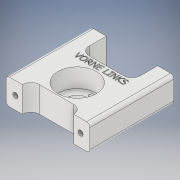
# Autodesk Inventor part: Motorhalterung leicht VL
Saved by Autodesk Inventor 2018 (Build 220112000, 112)
## iProperties
Created: 2019-03-03
Part Number: Motorhalterung leicht VL
Material: ABS-Kunststoff
Document SubType Name: Modeling
Designer: RedBots
Density: 0.513105 g/cm^3
Appearance: Weiß
Mass: 11 g
Surface Area: 84.958 cm^2
Volume: 21.4381 cm^3
Author: RedBots
Autodesk Inventor part; units mm, degrees
ref_plane "YZ Plane" through (0, 0, 0) normal (1, 0, 0) x (0, 1, 0)
ref_plane "XZ Plane" through (0, 0, 0) normal (0, 1, 0) x (-1, 0, 0)
ref_plane "XY Plane" through (0, 0, 0) normal (0, 0, 1) x (1, 0, 0)
sketch "Skizze2" plane through (0, 0, 0) normal (0, 0, 1) x (1, 0, 0)
  line L0 (0, 0) -> (49, 0)
  line L1 (0, 0) -> (49, 0) construction
  line L2 (49, 0) -> (49, 49)
  line L3 (49, 49) -> (0, 49)
  line L4 (0, 49) -> (0, 0)
  dimension "d16" = 49
  dimension "d18" = 49
  constraints: 10 end point, 2 equal length, 2 horizontal, 2 perpendicular
  measures "d16" distance of L0.start L0.end
  measures "d18" distance of L0.end L2.end
extrude "Extrusion1" add sketch "Skizze2" along normal blind 15
sketch "Skizze3" plane through (0, 0, 15) normal (0, 0, 1) x (1, 0, 0)
  circle A0 centre (24.5, 17) radius 11.25
  line L0 (0, 49) -> (0, 0) construction
  line L1 (0, 17) -> (49, 17) construction
  line L2 (49, 0) -> (49, 49) construction
  line L3 (0, 0) -> (49, 0) construction
  dimension "d72" = 22.5
  dimension "d73" = 17
  constraints: 2 end point, 2 point on line, 1 centre point, 1 coincident, 1 horizontal, 1 midpoint
  measures "d72" diameter of A0
  measures "d73" distance between parallel lines of L3 L1
extrude "Extrusion2" cut sketch "Skizze3" against normal blind 11
sketch "Skizze4" plane through (24.5, 17, 4) normal (0, 0, 1) x (1, 0, 0)
  circle A0 centre (7.3612, -4.25) radius 1.5
  circle A1 centre (0, 8.5) radius 1.5
  circle A2 centre (-7.3612, -4.25) radius 1.5
  line L0 (0, 0) -> (0, 8.5) construction
  line L1 (-24.5, -17) -> (24.5, -17) construction
  circle A3 centre (0, 0) radius 11.25 construction
  line L2 (0, -17) -> (0, 0) construction
  line L3 (0, 0) -> (7.3612, -4.25) construction
  line L4 (0, 0) -> (-7.3612, -4.25) construction
  circle A4 centre (0, 0) radius 6.5
  dimension "d37" = 3
  dimension "d42" = 3
  dimension "d43" = 3
  dimension "d90" = 8.5
  dimension "d91" = 120
  dimension "d92" = 120
  dimension "d93" = 13
  constraints: 8 end point, 4 centre point, 4 coincident, 2 equal length, 2 vertical, 1 midpoint
  measures "d37" diameter of A0
  measures "d42" diameter of A1
  measures "d43" diameter of A2
  measures "d90" distance of L0.start L0.end
  measures "d91" angle of L3 L0
  measures "d92" angle of L0 L4
  measures "d93" diameter of A4
extrude "Extrusion3" cut sketch "Skizze4" against normal up to next
sketch "Skizze9" plane through (0, 49, 0) normal (0, 1, 0) x (1, 0, 0)
  line L0 (24.5, -7.5) -> (43.5, -7.5) construction
  circle A0 centre (5.5, -7.5) radius 1.5
  circle A1 centre (43.5, -7.5) radius 1.5
  line L1 (0, -15) -> (49, -15) construction
  line L2 (24.5, -15) -> (24.5, 0) construction
  line L3 (49, 0) -> (0, 0) construction
  line L4 (5.5, -7.5) -> (24.5, -7.5) construction
  dimension "d58" = 3
  dimension "d89" = 19
  constraints: 7 end point, 3 midpoint, 2 centre point, 2 collinear, 1 coincident, 1 equal radius, 1 horizontal, 1 vertical
  measures "d58" diameter of A0
  measures "d89" distance of L0.start L0.end
extrude "Extrusion6" cut sketch "Skizze9" against normal blind 56
sketch "Skizze12" plane through (0, 0, 0) normal (0, 0, -1) x (-1, 0, 0)
  circle A0 centre (-24.5, 25.5) radius 1.5 projected
  circle A1 centre (-24.5, 25.5) radius 3
  circle A2 centre (-17.1388, 12.75) radius 1.5 projected
  circle A3 centre (-17.1388, 12.75) radius 3
  circle A4 centre (-31.8612, 12.75) radius 1.5 projected
  circle A5 centre (-31.8612, 12.75) radius 3
  point P0 (0, 0)
  dimension "d80" = 6
  dimension "d81" = 6
  dimension "d82" = 6
  constraints: 3 centre point, 3 coincident
  measures "d80" diameter of A1
  measures "d81" diameter of A3
  measures "d82" diameter of A5
extrude "Extrusion8" cut sketch "Skizze12" against normal blind 0.16
chamfer "Fase3" distance 1.5 angle 45 3 edges at (23, 25.5, 0.16) (30.3612, 12.75, 0.16) (15.6388, 12.75, 0.16)
fillet "Rundung2" radius 0.5 3 edges at (23, 25.5, 1.66) (30.3612, 12.75, 1.66) (15.6388, 12.75, 1.66)
sketch "Skizze14" plane through (0, 0, 0) normal (0, 0, -1) x (-1, 0, 0)
  line L0 (-39.5, 49) -> (-9.5, 49)
  line L1 (-9.5, 49) -> (-9.5, 34)
  line L2 (-9.5, 34) -> (-39.5, 34)
  line L3 (-39.5, 34) -> (-39.5, 49)
  line L4 (-49, 49) -> (0, 49) projected
  line L5 (-49, 0) -> (-49, 49) construction
  line L6 (0, 49) -> (0, 0) construction
  line L7 (-39.5, 0) -> (-9.5, 0)
  line L8 (-9.5, 0) -> (-9.5, 5)
  line L9 (-9.5, 5) -> (-39.5, 5)
  line L10 (-39.5, 5) -> (-39.5, 0)
  line L11 (0, 0) -> (-49, 0) projected
  point P0 (-24.5, 49)
  point P1 (-24.5, 0)
  point P2 (-24.5, 0)
  dimension "d95" = 15
  dimension "d96" = 30
  dimension "d101" = 5
  constraints: 16 end point, 6 midpoint, 3 horizontal, 3 parallel, 2 vertical, 1 perpendicular
  measures "d95" distance of L0.end L1.end
  measures "d96" distance between parallel lines of L1 L3
  measures "d101" distance of L7.end L9.start
extrude "Extrusion9" cut sketch "Skizze14" against normal up to next
fillet "Rundung3" radius 5 4 edges at (39.5, 34, 7.5) (9.5, 34, 7.5) (39.5, 5, 7.5) (9.5, 5, 7.5)
fillet "Rundung4" radius 2 4 edges at (49, 24.5, 15) (49, 24.5, 0) (0, 24.5, 0) (0, 24.5, 15)
sketch "Skizze15" plane through (0, 0, 15) normal (0, 0, 1) x (1, 0, 0)
  line L0 (34.5, 34) -> (14.5, 34) construction
  line L1 (24.5, 34) -> (24.5, 28.25) construction
  circle A0 centre (24.5, 17) radius 11.25 construction
  line L2 (12.5946, 32.875) -> (11.3892, 29.375)
  line L3 (11.3892, 29.375) -> (10.8872, 29.375)
  line L4 (10.8872, 29.375) -> (9.6817, 32.875)
  line L5 (9.6817, 32.875) -> (10.1809, 32.875)
  line L6 (10.1809, 32.875) -> (11.1509, 29.9678)
  line L7 (11.1509, 29.9678) -> (12.1209, 32.875)
  line L8 (12.1209, 32.875) -> (12.5946, 32.875)
  spline S0 degree 2 poles (15.4054, 32.4751) (15.6039, 32.2425) (15.8252, 31.5618) (15.8252, 31.125) knots 0 0 0 1 2 2 2
  spline S1 degree 2 poles (15.8252, 31.125) (15.8252, 30.6996) (15.6096, 30.0103) (15.4054, 29.7778) knots 0 0 0 1 2 2 2
  spline S2 degree 2 poles (15.4054, 29.7778) (15.1898, 29.5338) (14.6197, 29.3013) (14.2765, 29.3013) knots 0 0 0 1 2 2 2
  spline S3 degree 2 poles (14.2765, 29.3013) (13.922, 29.3013) (13.3547, 29.5423) (13.1477, 29.7778) knots 0 0 0 1 2 2 2
  spline S4 degree 2 poles (13.1477, 29.7778) (12.9463, 30.0103) (12.7308, 30.6939) (12.7308, 31.125) knots 0 0 0 1 2 2 2
  spline S5 degree 2 poles (12.7308, 31.125) (12.7308, 31.5646) (12.9491, 32.234) (13.1505, 32.4751) knots 0 0 0 1 2 2 2
  spline S6 degree 2 poles (13.1505, 32.4751) (13.3547, 32.7077) (13.9248, 32.9487) (14.2765, 32.9487) knots 0 0 0 1 2 2 2
  spline S7 degree 2 poles (14.2765, 32.9487) (14.6339, 32.9487) (15.2068, 32.6991) (15.4054, 32.4751) knots 0 0 0 1 2 2 2
  spline S8 degree 2 poles (15.3402, 31.125) (15.3402, 31.471) (15.1898, 32.0071) (15.0537, 32.1829) knots 0 0 0 1 2 2 2
  spline S9 degree 2 poles (15.0537, 32.1829) (14.9147, 32.3645) (14.5233, 32.546) (14.2794, 32.546) knots 0 0 0 1 2 2 2
  spline S10 degree 2 poles (14.2794, 32.546) (14.0269, 32.546) (13.6469, 32.3701) (13.5022, 32.1829) knots 0 0 0 1 2 2 2
  spline S11 degree 2 poles (13.5022, 32.1829) (13.3632, 32.0043) (13.2158, 31.4654) (13.2158, 31.125) knots 0 0 0 1 2 2 2
  spline S12 degree 2 poles (13.2158, 31.125) (13.2158, 30.4358) (13.7944, 29.704) (14.2794, 29.704) knots 0 0 0 1 2 2 2
  spline S13 degree 2 poles (14.2794, 29.704) (14.7644, 29.704) (15.3402, 30.4358) (15.3402, 31.125) knots 0 0 0 1 2 2 2
  line L9 (19.0444, 29.375) -> (18.4402, 29.375)
  line L10 (18.4402, 29.375) -> (17.3341, 30.7676)
  line L11 (17.3341, 30.7676) -> (16.8008, 30.7676)
  line L12 (16.8008, 30.7676) -> (16.8008, 29.375)
  line L13 (16.8008, 29.375) -> (16.3357, 29.375)
  line L14 (16.3357, 29.375) -> (16.3357, 32.875)
  line L15 (16.3357, 32.875) -> (17.2376, 32.875)
  spline S14 degree 2 poles (17.2376, 32.875) (17.5383, 32.875) (17.9439, 32.8098) (18.1282, 32.6906) knots 0 0 0 1 2 2 2
  spline S15 degree 2 poles (18.1282, 32.6906) (18.3126, 32.5715) (18.5253, 32.2) (18.5253, 31.9248) knots 0 0 0 1 2 2 2
  spline S16 degree 2 poles (18.5253, 31.9248) (18.5253, 31.5419) (18.1339, 31.0229) (17.7992, 30.8981) knots 0 0 0 1 2 2 2
  line L16 (17.7992, 30.8981) -> (19.0444, 29.375)
  spline S17 degree 2 poles (18.0403, 31.888) (18.0403, 32.0411) (17.9325, 32.2765) (17.8191, 32.3531) knots 0 0 0 1 2 2 2
  spline S18 degree 2 poles (17.8191, 32.3531) (17.7198, 32.4184) (17.456, 32.4722) (17.2632, 32.4722) knots 0 0 0 1 2 2 2
  line L17 (17.2632, 32.4722) -> (16.8008, 32.4722)
  line L18 (16.8008, 32.4722) -> (16.8008, 31.1562)
  line L19 (16.8008, 31.1562) -> (17.2093, 31.1562)
  spline S19 degree 2 poles (17.2093, 31.1562) (17.4107, 31.1562) (17.7312, 31.2271) (17.8418, 31.3377) knots 0 0 0 1 2 2 2
  spline S20 degree 2 poles (17.8418, 31.3377) (17.9439, 31.4342) (18.0403, 31.7064) (18.0403, 31.888) knots 0 0 0 1 2 2 2
  line L20 (21.8268, 29.375) -> (21.3049, 29.375)
  line L21 (21.3049, 29.375) -> (19.7563, 32.3928)
  line L22 (19.7563, 32.3928) -> (19.7563, 29.375)
  line L23 (19.7563, 29.375) -> (19.3223, 29.375)
  line L24 (19.3223, 29.375) -> (19.3223, 32.875)
  line L25 (19.3223, 32.875) -> (19.9832, 32.875)
  line L26 (19.9832, 32.875) -> (21.3928, 30.1039)
  line L27 (21.3928, 30.1039) -> (21.3928, 32.875)
  line L28 (21.3928, 32.875) -> (21.8268, 32.875)
  line L29 (21.8268, 32.875) -> (21.8268, 29.375)
  line L30 (22.5359, 29.375) -> (22.5359, 32.875)
  line L31 (22.5359, 32.875) -> (24.7255, 32.875)
  line L32 (24.7255, 32.875) -> (24.7255, 32.4609)
  line L33 (24.7255, 32.4609) -> (23.001, 32.4609)
  line L34 (23.001, 32.4609) -> (23.001, 31.5022)
  line L35 (23.001, 31.5022) -> (24.6092, 31.5022)
  line L36 (24.6092, 31.5022) -> (24.6092, 31.0881)
  line L37 (24.6092, 31.0881) -> (23.001, 31.0881)
  line L38 (23.001, 31.0881) -> (23.001, 29.7891)
  line L39 (23.001, 29.7891) -> (24.7255, 29.7891)
  line L40 (24.7255, 29.7891) -> (24.7255, 29.375)
  line L41 (24.7255, 29.375) -> (22.5359, 29.375)
  line L42 (28.7672, 29.375) -> (26.7393, 29.375)
  line L43 (26.7393, 29.375) -> (26.7393, 32.875)
  line L44 (26.7393, 32.875) -> (27.2044, 32.875)
  line L45 (27.2044, 32.875) -> (27.2044, 29.7891)
  line L46 (27.2044, 29.7891) -> (28.7672, 29.7891)
  line L47 (28.7672, 29.7891) -> (28.7672, 29.375)
  line L48 (30.3527, 29.375) -> (28.997, 29.375)
  line L49 (28.997, 29.375) -> (28.997, 29.7324)
  line L50 (28.997, 29.7324) -> (29.4423, 29.7324)
  line L51 (29.4423, 29.7324) -> (29.4423, 32.5176)
  line L52 (29.4423, 32.5176) -> (28.997, 32.5176)
  line L53 (28.997, 32.5176) -> (28.997, 32.875)
  line L54 (28.997, 32.875) -> (30.3527, 32.875)
  line L55 (30.3527, 32.875) -> (30.3527, 32.5176)
  line L56 (30.3527, 32.5176) -> (29.9074, 32.5176)
  line L57 (29.9074, 32.5176) -> (29.9074, 29.7324)
  line L58 (29.9074, 29.7324) -> (30.3527, 29.7324)
  line L59 (30.3527, 29.7324) -> (30.3527, 29.375)
  line L60 (33.4329, 29.375) -> (32.9111, 29.375)
  line L61 (32.9111, 29.375) -> (31.3624, 32.3928)
  line L62 (31.3624, 32.3928) -> (31.3624, 29.375)
  line L63 (31.3624, 29.375) -> (30.9285, 29.375)
  line L64 (30.9285, 29.375) -> (30.9285, 32.875)
  line L65 (30.9285, 32.875) -> (31.5893, 32.875)
  line L66 (31.5893, 32.875) -> (32.999, 30.1039)
  line L67 (32.999, 30.1039) -> (32.999, 32.875)
  line L68 (32.999, 32.875) -> (33.4329, 32.875)
  line L69 (33.4329, 32.875) -> (33.4329, 29.375)
  line L70 (36.6947, 29.375) -> (36.0906, 29.375)
  line L71 (36.0906, 29.375) -> (34.8114, 31.003)
  line L72 (34.8114, 31.003) -> (34.6072, 30.7733)
  line L73 (34.6072, 30.7733) -> (34.6072, 29.375)
  line L74 (34.6072, 29.375) -> (34.142, 29.375)
  line L75 (34.142, 29.375) -> (34.142, 32.875)
  line L76 (34.142, 32.875) -> (34.6072, 32.875)
  line L77 (34.6072, 32.875) -> (34.6072, 31.2668)
  line L78 (34.6072, 31.2668) -> (36.0423, 32.875)
  line L79 (36.0423, 32.875) -> (36.6096, 32.875)
  line L80 (36.6096, 32.875) -> (35.1602, 31.3122)
  line L81 (35.1602, 31.3122) -> (36.6947, 29.375)
  spline S21 degree 2 poles (37.9483, 29.3126) (37.5683, 29.3126) (37.035, 29.4714) (36.7996, 29.5849) knots 0 0 0 1 2 2 2
  line L82 (36.7996, 29.5849) -> (36.7996, 30.1692)
  line L83 (36.7996, 30.1692) -> (36.8337, 30.1692)
  spline S22 degree 2 poles (36.8337, 30.1692) (37.0634, 29.9536) (37.6449, 29.7154) (37.9143, 29.7154) knots 0 0 0 1 2 2 2
  spline S23 degree 2 poles (37.9143, 29.7154) (38.3, 29.7154) (38.6943, 30.0359) (38.6943, 30.2996) knots 0 0 0 1 2 2 2
  spline S24 degree 2 poles (38.6943, 30.2996) (38.6943, 30.5095) (38.4872, 30.7705) (38.2632, 30.8357) knots 0 0 0 1 2 2 2
  spline S25 degree 2 poles (38.2632, 30.8357) (38.1015, 30.8811) (37.832, 30.9435) (37.6307, 30.9945) knots 0 0 0 1 2 2 2
  spline S26 degree 2 poles (37.6307, 30.9945) (37.4491, 31.0427) (37.1627, 31.1874) (37.0521, 31.3037) knots 0 0 0 1 2 2 2
  spline S27 degree 2 poles (37.0521, 31.3037) (36.9443, 31.42) (36.8252, 31.732) (36.8252, 31.9362) knots 0 0 0 1 2 2 2
  spline S28 degree 2 poles (36.8252, 31.9362) (36.8252, 32.3616) (37.4889, 32.9374) (38.0022, 32.9374) knots 0 0 0 1 2 2 2
  spline S29 degree 2 poles (38.0022, 32.9374) (38.2972, 32.9374) (38.8191, 32.8211) (39.0432, 32.7105) knots 0 0 0 1 2 2 2
  line L84 (39.0432, 32.7105) -> (39.0432, 32.1546)
  line L85 (39.0432, 32.1546) -> (39.0091, 32.1546)
  spline S30 degree 2 poles (39.0091, 32.1546) (38.8418, 32.3077) (38.3199, 32.5346) (38.0334, 32.5346) knots 0 0 0 1 2 2 2
  spline S31 degree 2 poles (38.0334, 32.5346) (37.7101, 32.5346) (37.3102, 32.2312) (37.3102, 31.9844) knots 0 0 0 1 2 2 2
  spline S32 degree 2 poles (37.3102, 31.9844) (37.3102, 31.7632) (37.5456, 31.4994) (37.7668, 31.4398) knots 0 0 0 1 2 2 2
  spline S33 degree 2 poles (37.7668, 31.4398) (37.9143, 31.4001) (38.3426, 31.298) (38.4844, 31.2555) knots 0 0 0 1 2 2 2
  spline S34 degree 2 poles (38.4844, 31.2555) (38.8446, 31.1449) (39.1793, 30.6996) (39.1793, 30.3734) knots 0 0 0 1 2 2 2
  spline S35 degree 2 poles (39.1793, 30.3734) (39.1793, 30.1663) (39.012, 29.7692) (38.8616, 29.6303) knots 0 0 0 1 2 2 2
  spline S36 degree 2 poles (38.8616, 29.6303) (38.6943, 29.4771) (38.2688, 29.3126) (37.9483, 29.3126) knots 0 0 0 1 2 2 2
  point P0 (0, 0)
  point P1 (24.5, 31.125)
  point P2 (24.5, 31.125)
  constraints: 2 end point, 2 midpoint, 1 coincident, 1 vertical alignment, 2 other
emboss "Prägen1" sketch "Skizze15" operation cut depth 1 direction (0, 0, -1)
